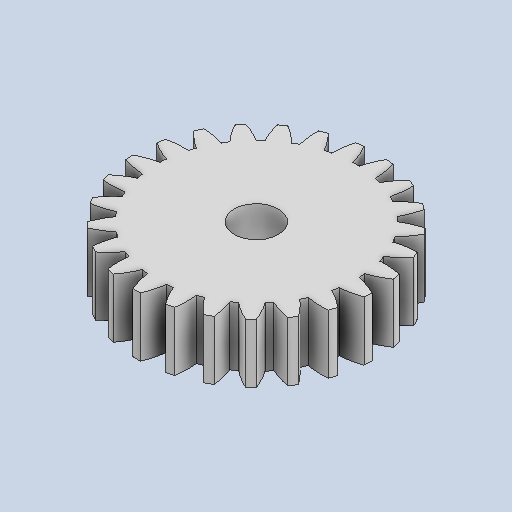
# Autodesk Inventor part: pinion_source_25
Saved by Autodesk Inventor 2022 (Build 260153000, 153)
## iProperties
Created: 2022-07-22
Part Number: pinion_source_25
Material: 一般
Document SubType Name: Modeling
Designer: Yazawa
Density: 1 g/cm^3
Appearance: 既定
Author: Yazawa
Autodesk Inventor part; units mm, degrees
ref_plane "YZ Plane" through (0, 0, 0) normal (1, 0, 0) x (0, 1, 0)
ref_plane "XZ Plane" through (0, 0, 0) normal (0, 1, 0) x (-1, 0, 0)
ref_plane "XY Plane" through (0, 0, 0) normal (0, 0, 1) x (1, 0, 0)
sketch "スケッチ1" plane through (0, 0, 0) normal (0, 1, 0) x (-1, 0, 0)
  circle A0 centre (0, 0) radius 4.05
  circle A1 centre (0, 0) radius 0.75
  dimension "d0" = 8.1
  dimension "d1" = 1.5
  constraints: 2 centre point, 2 coincident
  measures "d0" diameter of A0
  measures "d1" diameter of A1
extrude "押し出し1" add sketch "スケッチ1" along normal blind 2
spur gear teeth "平歯車1" teeth 25 pitch diameter 7.5 tip diameter 8.1009 root diameter 6.7509 face width 2 trims to tip circle yes start plane through (0, 0, 0) normal (0, -1, 0) x (1, 0, 0)
